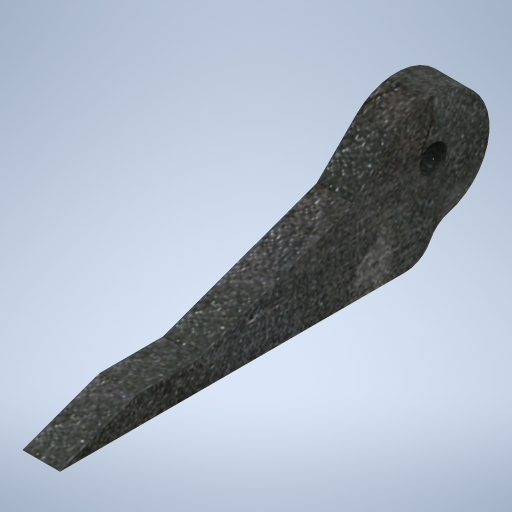
# Autodesk Inventor part: Wedgelet
Saved by Autodesk Inventor 2023 (Build 270158000, 158)
## iProperties
Created: 2023-01-30
Part Number: Wedgelet
Material: Steel
Document SubType Name: Modeling
Designer: justi
Density: 7.85 g/cm^3
Appearance: Plate
Author: justi
Autodesk Inventor part; units mm, degrees
ref_plane "YZ Plane" through (0, 0, 0) normal (1, 0, 0) x (0, 1, 0)
ref_plane "XZ Plane" through (0, 0, 0) normal (0, 1, 0) x (-1, 0, 0)
ref_plane "XY Plane" through (0, 0, 0) normal (0, 0, 1) x (1, 0, 0)
sketch "Sketch1" plane through (0, 0, 0) normal (1, 0, 0) x (0, 1, 0)
  circle A0 centre (0, 0) radius 4.7625
  circle A1 centre (0, 0) radius 19.05
  dimension "d0" = 9.525
  dimension "d1" = 38.1
  constraints: 2 centre point, 2 coincident
  measures "d0" diameter of A0
  measures "d1" diameter of A1
extrude "Extrusion1" add sketch "Sketch1" along normal blind 12.7
sketch "Sketch2" plane through (12.7, 0, 0) normal (1, 0, 0) x (0, 0, -1)
  circle A0 centre (0, 0) radius 19.05 projected
  line L0 (0, -19.05) -> (-50.8, -19.05)
  circle A1 centre (0, 0) radius 4.7625 projected
  line L1 (0, -19.05) -> (11.4002, -19.05)
  line L2 (-13.4704, 13.4704) -> (-25.8301, 1.1106)
  line L3 (0, 0) -> (-13.4704, 13.4704)
  line L4 (0, 0) -> (-19.05, 0)
  line L5 (-25.8301, 1.1106) -> (-26.9408, 0)
  line L6 (0, -19.05) -> (-127, -19.05)
  line L7 (0, -38.1) -> (0, -19.05)
  line L8 (-26.9408, 0) -> (-59.9363, -19.05)
  line L9 (0, -28.575) -> (-127, -28.575)
  line L10 (-127, -28.575) -> (-100.8303, -19.05)
  line L11 (-79.2802, -19.05) -> (16.9609, 15.9789)
  dimension "d6" = 50.8
  dimension "d7" = 0
  dimension "d8" = 180
  dimension "d9" = 45
  dimension "d10" = 45
  dimension "d11" = 17.4793
  dimension "d13" = 19.05
  dimension "d17" = 30
  dimension "d18" = 180
  dimension "d19" = 38.1
  dimension "d20" = 127
  dimension "d21" = 20
  dimension "d24" = 20
  dimension "d25" = 0
  constraints: 24 end point, 4 horizontal, 4 point on circle, 3 point on line, 1 midpoint
  measures "d6" distance of L0.start L0.end
  measures "d7" horizontal distance of L3.start L0.start
  measures "d8" angle of L0 L1
  measures "d9" angle of L3 L4
  measures "d10" angle of L4 L2
  measures "d11" distance of L2.start L2.end
  measures "d13" distance of L7.start L1.start
  measures "d17" angle of L0 L8
  measures "d18" angle of L5 L2
  measures "d19" distance of L5.end L8.end
  measures "d20" distance of L9.start L9.end
  measures "d21" angle of L9 L10
  measures "d24" angle of L6 L11
  measures "d25" distance from line of L5.end L11
extrude "Extrusion2" add sketch "Sketch2" against normal blind 12.7 contours A0 L0 L6 L8 L11 | L7 L9 L10 L6 L0 | L11 L5 L2 A0
sketch "Sketch3" plane through (12.7, 0, 0) normal (1, 0, 0) x (0, 0, -1)
  line L0 (-59.9363, -19.05) -> (-26.9408, 0) projected
  line L1 (-26.9408, 0) -> (-79.2802, -19.05)
  line L2 (-100.8303, -19.05) -> (-59.9363, -19.05) projected
  line L3 (-79.2802, -19.05) -> (-59.9363, -19.05)
  line L4 (-26.9408, 0) -> (-59.9363, -19.05)
  point P0 (0, 0)
  dimension "d26" = 20
  constraints: 6 end point, 2 collinear, 1 point on line
  measures "d26" angle of L2 L1
extrude "Extrusion3" add sketch "Sketch3" against normal blind 12.7
fillet "Fillet1" radius 9.525 1 edges at (6.35, -28.575, 0)
fillet "Fillet2" radius 9.525 2 edges at (6.35, -19.0505, 0) (6.35, -19.05, 0)
sketch "Sketch4" plane through (12.7, 0, 0) normal (1, 0, 0) x (0, 0, -1)
  point P0 (0, 0)
body "Solid1"
